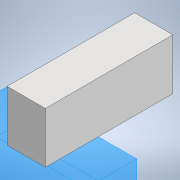
# Autodesk Inventor part: XLimit OffsetBlock
Saved by Autodesk Inventor 2020 (Build 240168000, 168)
## iProperties
Created: 2019-09-14
Part Number: XLimit OffsetBlock
Material: Generic
Document SubType Name: Modeling
Designer: pepd9
Density: 1 g/cm^3
Appearance: Default
Author: pepd9
Autodesk Inventor part; units mm, degrees
ref_plane "YZ Plane" through (0, 0, 0) normal (1, 0, 0) x (0, 1, 0)
ref_plane "XZ Plane" through (0, 0, 0) normal (0, 1, 0) x (-1, 0, 0)
ref_plane "XY Plane" through (0, 0, 0) normal (0, 0, 1) x (1, 0, 0)
sketch "Sketch1" plane through (0, 0, 0) normal (0, 0, 1) x (1, 0, 0)
  line L0 (-17.0171, 4) -> (-11.0171, 4)
  line L1 (-11.0171, 4) -> (-11.0171, -4)
  line L2 (-11.0171, -4) -> (-17.0171, -4)
  line L3 (-17.0171, -4) -> (-17.0171, 4)
  line L4 (-17.0171, 4) -> (-11.0171, -4) construction
  line L5 (-11.0171, 4) -> (-17.0171, -4) construction
  point P0 (0, 0)
  point P1 (-14.0171, 0)
  dimension "d0" = 6
  dimension "d1" = 8
  constraints: 12 end point, 2 midpoint, 2 parallel, 1 horizontal, 1 perpendicular
  measures "d0" distance of L1.end L2.end
  measures "d1" distance of L0.end L1.end
extrude "Extrusion1" add sketch "Sketch1" along normal blind 20
body "Solid1"
